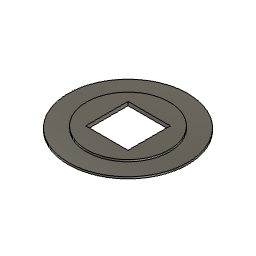
separator (Autodesk Fusion 360 design; units mm, degrees)
Autodesk Fusion 360 part; units mm, degrees
sketch "Sketch1" plane through (0, 0, 0) normal (0, 0, 1) x (1, 0, 0)
  circle A0 centre (0, 0) radius 32.5
  line L0 (-11.5, 11.5) -> (11.5, 11.5)
  line L1 (11.5, 11.5) -> (11.5, -11.5)
  line L2 (11.5, -11.5) -> (-11.5, -11.5)
  line L3 (-11.5, -11.5) -> (-11.5, 11.5)
  point P0 (11.5, 0)
  point P1 (0, 11.5)
  dimension "d1" = 65
  dimension "d2" = 23
  constraint coincident A0.centre origin
  constraint horizontal L0
  constraint vertical L1
  constraint horizontal L2
  constraint vertical L3
  constraint midpoint L1 P0
  constraint midpoint L0 P1
  constraint vertical A0.centre P1
  constraint horizontal A0.centre P0
  constraint equal L0 L3
  measures "d1" diameter of A0
  measures "d2" distance of L0.start L0.end
extrude "Extrude1" add sketch "Sketch1" along normal blind 1
sketch "Sketch2" plane through (0, 0, 1) normal (0, 0, 1) x (-1, 0, 0)
  line L0 (-11.5, 11.5) -> (11.5, 11.5)
  line L1 (11.5, 11.5) -> (11.5, -11.5)
  line L2 (11.5, -11.5) -> (-11.5, -11.5)
  line L3 (-11.5, -11.5) -> (-11.5, 11.5)
  circle A0 centre (0, 0) radius 32.5
  line L4 (11.5, -11.5) -> (-11.5, -11.5)
  line L5 (-11.5, -11.5) -> (-11.5, 11.5)
  line L6 (-11.5, 11.5) -> (11.5, 11.5)
  line L7 (11.5, 11.5) -> (11.5, -11.5)
  circle A1 centre (0, 0) radius 22.5
  dimension "d5" = 45
  constraint horizontal L4
  constraint vertical L5
  constraint horizontal L6
  constraint vertical L7
  constraint coincident L0.start L3.end
  constraint coincident L1.end L2.start
  constraint coincident A0.centre A1.centre
  measures "d5" diameter of A1
extrude "Extrude2" add sketch "Sketch2" along normal blind 1 contours A1
